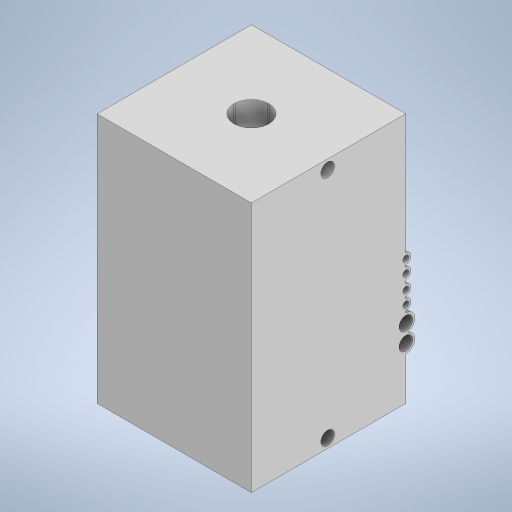
# Autodesk Inventor part: LightSensorHousing
Saved by Autodesk Inventor 2023 (Build 270158000, 158)
## iProperties
Created: 2023-07-05
Part Number: LightSensorHousing
Material: Generic
Document SubType Name: Modeling
Designer: efarq
Density: 1 g/cm^3
Appearance: Default
Author: efarq
Autodesk Inventor part; units mm, degrees
ref_plane "YZ Plane" through (0, 0, 0) normal (1, 0, 0) x (0, 1, 0)
ref_plane "XZ Plane" through (0, 0, 0) normal (0, 1, 0) x (-1, 0, 0)
ref_plane "XY Plane" through (0, 0, 0) normal (0, 0, 1) x (1, 0, 0)
sketch "Sketch1" plane through (0, 0, 0) normal (0, 0, 1) x (1, 0, 0)
  line L0 (-25.4, -41.275) -> (25.4, -41.275)
  line L1 (25.4, -41.275) -> (25.4, 41.275)
  line L2 (25.4, 41.275) -> (-25.4, 41.275)
  line L3 (-25.4, 41.275) -> (-25.4, -41.275)
  line L4 (-25.4, -41.275) -> (25.4, 41.275) construction
  line L5 (25.4, -41.275) -> (-25.4, 41.275) construction
  point P0 (0, 0)
  dimension "d0" = 50.8
  dimension "d1" = 82.55
  constraints: 12 end point, 2 midpoint, 2 parallel, 1 horizontal, 1 perpendicular
  measures "d0" distance of L2.end L1.end
  measures "d1" distance of L0.end L1.end
extrude "Extrusion1" add sketch "Sketch1" along normal blind 50.8
sketch "Sketch2" plane through (-25.4, 41.275, 0) normal (0, 1, 0) x (1, 0, 0)
  circle A0 centre (25.4, -25.4) radius 5.715
  line L0 (50.8, 0) -> (0, 0) projected
  point P0 (25.4, 0)
  dimension "d4" = 11.43
  dimension "d5" = 25.4
  constraints: 1 centre point
  measures "d4" diameter of A0
  measures "d5" distance from line of L0 A0.centre
extrude "Extrusion2" cut sketch "Sketch2" against normal blind 33.02
sketch "Sketch3" plane through (0, 0, 0) normal (0, 0, -1) x (-1, 0, 0)
  line L0 (-13.97, 8.255) -> (13.97, 8.255)
  line L1 (13.97, 8.255) -> (13.97, 28.575)
  line L2 (13.97, 28.575) -> (-13.97, 28.575)
  line L3 (-13.97, 28.575) -> (-13.97, 8.255)
  line L4 (-13.97, 8.255) -> (13.97, 28.575) construction
  line L5 (13.97, 8.255) -> (-13.97, 28.575) construction
  line L6 (-25.4, 41.275) -> (25.4, 41.275) projected
  line L7 (25.4, 41.275) -> (25.4, -41.275) projected
  point P0 (0, 0)
  point P1 (0, 18.415)
  dimension "d9" = 27.94
  dimension "d10" = 20.32
  dimension "d11" = 12.7
  dimension "d14" = 25.4
  constraints: 12 end point, 2 midpoint, 2 parallel, 1 horizontal, 1 perpendicular
  measures "d9" distance of L1.end L2.end
  measures "d10" distance of L0.end L1.end
  measures "d11" distance between parallel lines of L2 L6
  measures "d14" distance from line of L7 point (0, 18.415)
extrude "Extrusion3" cut sketch "Sketch3" against normal blind 19.304
sketch "Sketch6" plane through (0, 0, 19.304) normal (0, 0, -1) x (-1, 0, 0)
  line L0 (-13.97, 15.113) -> (-9.144, 15.113)
  line L1 (-9.144, 15.113) -> (-9.144, 21.717)
  line L2 (-9.144, 21.717) -> (-13.97, 21.717)
  line L3 (-13.97, 21.717) -> (-13.97, 15.113)
  line L4 (-13.97, 15.113) -> (-9.144, 21.717) construction
  line L5 (-9.144, 15.113) -> (-13.97, 21.717) construction
  line L6 (13.97, 28.575) -> (13.97, 8.255) projected
  line L7 (9.144, 15.113) -> (13.97, 15.113)
  line L8 (13.97, 15.113) -> (13.97, 21.717)
  line L9 (13.97, 21.717) -> (9.144, 21.717)
  line L10 (9.144, 21.717) -> (9.144, 15.113)
  line L11 (9.144, 15.113) -> (13.97, 21.717) construction
  line L12 (13.97, 15.113) -> (9.144, 21.717) construction
  line L13 (-13.97, 8.255) -> (-13.97, 28.575) projected
  line L14 (-13.97, 28.575) -> (13.97, 28.575) projected
  point P0 (0, 0)
  point P1 (-11.557, 18.415)
  point P2 (11.557, 18.415)
  point P3 (13.97, 15.113)
  dimension "d15" = 6.604
  dimension "d16" = 4.826
  dimension "d17" = 2.413
  dimension "d18" = 4.826
  dimension "d19" = 6.604
  dimension "d21" = 6.858
  dimension "d22" = 6.858
  constraints: 24 end point, 4 midpoint, 4 parallel, 2 horizontal, 2 perpendicular, 1 point on line
  measures "d15" distance of L0.end L1.end
  measures "d16" distance of L1.end L2.end
  measures "d17" distance from line of L13 point (-11.557, 18.415)
  measures "d18" distance of L8.end L9.end
  measures "d19" distance of L9.end L7.start
  measures "d21" distance between parallel lines of L9 L14
  measures "d22" distance between parallel lines of L14 L2
extrude "Extrusion4" cut sketch "Sketch6" against normal blind 4.826
sketch "Sketch7" plane through (0, 0, 19.304) normal (0, 0, -1) x (-1, 0, 0)
  line L0 (-2.3813, 16.0401) -> (2.3813, 16.0401)
  line L1 (2.3813, 16.0401) -> (2.3812, 20.8026)
  line L2 (2.3812, 20.8026) -> (-2.3813, 20.8026)
  line L3 (-2.3813, 20.8026) -> (-2.3813, 16.0401)
  line L4 (-2.3813, 16.0401) -> (2.3812, 20.8026) construction
  line L5 (2.3813, 16.0401) -> (-2.3813, 20.8026) construction
  line L6 (9.144, 15.113) -> (9.144, 21.717) projected
  line L7 (-13.97, 28.575) -> (13.97, 28.575) projected
  point P0 (0, 0)
  point P1 (0, 18.4213)
  point P2 (0, 20.8026)
  dimension "d25" = 4.7625
  dimension "d26" = 9.144
  dimension "d27" = 4.7625
  dimension "d29" = 7.7724
  constraints: 12 end point, 3 midpoint, 2 parallel, 1 horizontal, 1 perpendicular
  measures "d25" distance of L1.end L2.end
  measures "d26" distance from line of L6 point (0, 18.421)
  measures "d27" distance of L2.end L0.start
  measures "d29" distance from line of point (0, 20.803) L7
extrude "Extrusion5" cut sketch "Sketch7" against normal blind 4.826
sketch "Sketch8" plane through (-25.4, -41.275, 0) normal (-1, 0, 0) x (0, 0, 1)
  line L0 (15.24, 11.43) -> (35.56, 11.43)
  line L1 (35.56, 11.43) -> (35.56, 57.15)
  line L2 (35.56, 57.15) -> (15.24, 57.15)
  line L3 (15.24, 57.15) -> (15.24, 11.43)
  line L4 (15.24, 11.43) -> (35.56, 57.15) construction
  line L5 (35.56, 11.43) -> (15.24, 57.15) construction
  line L6 (50.8, 82.55) -> (50.8, 0) projected
  line L7 (0, 82.55) -> (50.8, 82.55) projected
  point P0 (0, 41.275)
  point P1 (25.4, 34.29)
  dimension "d32" = 45.72
  dimension "d33" = 20.32
  dimension "d34" = 25.4
  dimension "d35" = 25.4
  constraints: 12 end point, 2 midpoint, 2 parallel, 1 horizontal, 1 perpendicular
  measures "d32" distance of L0.end L1.end
  measures "d33" distance of L0.start L0.end
  measures "d34" distance from line of L6 point (25.4, 34.29)
  measures "d35" distance between parallel lines of L7 L2
extrude "Extrusion6" cut sketch "Sketch8" against normal blind 10.16
sketch "Sketch11" plane through (-25.4, -41.275, 0) normal (-1, 0, 0) x (0, 0, 1)
  circle A0 centre (27.4828, 60.96) radius 3.302
  line L0 (0, 82.55) -> (50.8, 82.55) projected
  line L1 (50.8, 82.55) -> (50.8, 0) projected
  point P0 (0, 41.275)
  dimension "d43" = 6.604
  dimension "d44" = 21.59
  dimension "d45" = 23.3172
  constraints: 1 centre point
  measures "d43" diameter of A0
  measures "d44" distance from line of A0.centre L0
  measures "d45" distance from line of L1 A0.centre
extrude "Extrusion7" cut sketch "Sketch11" against normal blind 25.4
sketch "Sketch14" plane through (-25.4, 41.275, 0) normal (0, 1, 0) x (1, 0, 0)
  line L0 (19.685, -31.115) -> (31.115, -31.115)
  line L1 (31.115, -31.115) -> (31.115, -19.685)
  line L2 (31.115, -19.685) -> (19.685, -19.685)
  line L3 (19.685, -19.685) -> (19.685, -31.115)
  circle A0 centre (25.4, -25.4) radius 5.715 projected
  line L4 (19.685, -31.115) -> (31.115, -19.685) construction
  line L5 (31.115, -31.115) -> (19.685, -19.685) construction
  point P0 (25.4, 0)
  constraints: 12 end point, 2 midpoint, 2 parallel, 1 horizontal, 1 perpendicular
extrude "Extrusion8" cut sketch "Sketch14" against normal blind 33.02
sketch "Sketch15" plane through (-25.4, 41.275, 0) normal (0, 1, 0) x (1, 0, 0)
  circle A0 centre (25.4, -25.4) radius 5.725
  line L0 (31.115, -19.685) -> (31.115, -31.115) projected
  line L1 (19.685, -19.685) -> (31.115, -19.685)
  line L2 (31.115, -19.685) -> (31.115, -31.115)
  line L3 (31.115, -31.115) -> (19.685, -31.115)
  line L4 (19.685, -31.115) -> (19.685, -19.685)
  line L5 (19.685, -19.685) -> (31.115, -31.115) construction
  line L6 (31.115, -19.685) -> (19.685, -31.115) construction
  point P0 (25.4, 0)
  point P1 (19.685, -25.0617)
  point P2 (25.0617, -19.685)
  point P3 (25.7383, -19.685)
  point P4 (31.115, -25.0617)
  point P5 (19.685, -25.7383)
  point P6 (25.0617, -31.115)
  point P7 (25.7383, -31.115)
  point P8 (31.115, -25.7383)
  constraints: 12 end point, 2 midpoint, 2 parallel, 1 centre point, 1 horizontal, 1 perpendicular
extrude "Extrusion9" add sketch "Sketch15" against normal blind 10.16 contours A0 L1 L0 | L0 L3 A0 | A0 L4 L1 | L3 L4 A0
sketch "Sketch16" plane through (-25.4, 15.875, 15.24) normal (0, -1, 0) x (1, 0, 0)
  circle A0 centre (2.2186, 12.8252) radius 0.4886
  circle A1 centre (2.2186, 11.3059) radius 0.4826
  line L0 (11.43, 4.064) -> (11.43, 8.89) projected
  point P0 (25.4, -15.24)
  dimension "d57" = 0.9772
  dimension "d59" = 0.9652
  constraints: 2 centre point
  measures "d57" diameter of A0
  measures "d59" diameter of A1
extrude "Extrusion10" cut sketch "Sketch16" against normal blind 2.54
sketch "Sketch17" plane through (25.4, -41.275, 0) normal (1, 0, 0) x (0, 0, -1)
  line L0 (-25.7383, 82.55) -> (-25.7383, 72.39) projected
  circle A0 centre (-25.7383, 79.502) radius 2.2209
  circle A1 centre (-25.7383, 3.048) radius 2.2225
  line L1 (0, 82.55) -> (-50.8, 82.55) projected
  line L2 (0, 0) -> (-50.8, 0) projected
  point P0 (0, 41.275)
  dimension "d62" = 4.4418
  dimension "d63" = 4.445
  dimension "d64" = 3.048
  dimension "d65" = 3.048
  constraints: 2 centre point, 1 point on line
  measures "d62" diameter of A0
  measures "d63" diameter of A1
  measures "d64" distance from line of L1 A0.centre
  measures "d65" distance from line of L2 A1.centre
extrude "Extrusion11" cut sketch "Sketch17" against normal blind 7
sketch "Sketch18" plane through (25.4, -41.275, 0) normal (1, 0, 0) x (0, 0, -1)
  line L0 (0, 0) -> (0, 82.55) projected
  circle A0 centre (0, 41.275) radius 1.75
  point P0 (0, 41.275)
  dimension "d71" = 3.5
  constraints: 1 centre point, 1 coincident, 1 midpoint
  measures "d71" diameter of A0
extrude "Extrusion12" add sketch "Sketch18" against normal blind 16.5
sketch "Sketch19" plane through (-13.97, 8.255, 0) normal (0, 1, 0) x (1, 0, 0)
  line L0 (0, 0) -> (27.94, 0) projected
  circle A0 centre (24.62, 0) radius 1.75
  line L1 (22.87, 1.75) -> (22.87, 0) projected
  point P0 (13.97, 0)
  dimension "d77" = 3.5
  dimension "d78" = 1.75
  constraints: 1 centre point, 1 point on line
  measures "d77" diameter of A0
  measures "d78" distance from line of L1 A0.centre
extrude "Extrusion13" add sketch "Sketch19" against normal blind 8
sketch "Sketch20" plane through (25.4, -41.275, 50.8) normal (1, 0, 0) x (0, 0, -1)
  circle A0 centre (50.8, 41.275) radius 1
  dimension "d81" = 2
  constraints: 1 centre point, 1 coincident
  measures "d81" diameter of A0
extrude "Extrusion14" cut sketch "Sketch20" against normal blind 16
sketch "Sketch21" plane through (-13.97, 8.255, 19.304) normal (0, 1, 0) x (1, 0, 0)
  circle A0 centre (24.6331, 19.304) radius 1
  arc A1 (26.37, 19.304) -> (22.87, 19.304) centre (24.62, 19.304) ccw projected
  point P0 (13.97, 19.304)
  dimension "d84" = 2
  constraints: 1 centre point
  measures "d84" diameter of A0
extrude "Extrusion15" cut sketch "Sketch21" against normal blind 8.5
sketch "Sketch22" plane through (25.4, -41.275, 50.8) normal (1, 0, 0) x (0, 0, -1)
  line L0 (50.8, 82.55) -> (50.8, 0) projected
  circle A0 centre (50.8, 37.084) radius 1.75
  point P0 (50.8, 41.275)
  point P1 (50.8, 41.275)
  dimension "d88" = 3.5
  dimension "d89" = 4.191
  constraints: 1 centre point, 1 midpoint, 1 point on line
  measures "d88" diameter of A0
  measures "d89" distance of A0.centre point (50.8, 41.275)
extrude "Extrusion16" add sketch "Sketch22" against normal blind 20.75
sketch "Sketch23" plane through (-13.97, 8.255, 19.304) normal (0, 1, 0) x (1, 0, 0)
  line L0 (0, 19.304) -> (22.87, 19.304) projected
  circle A0 centre (20.429, 19.304) radius 1.75
  arc A1 (26.37, 19.304) -> (22.87, 19.304) centre (24.62, 19.304) ccw projected
  point P0 (13.97, 19.304)
  dimension "d92" = 3.5
  dimension "d93" = 4.191
  constraints: 1 centre point, 1 point on line
  measures "d92" diameter of A0
  measures "d93" distance of A1.centre A0.centre
extrude "Extrusion17" add sketch "Sketch23" against normal blind 12
sketch "Sketch24" plane through (-13.97, 8.255, 19.304) normal (0, 1, 0) x (1, 0, 0)
  circle A0 centre (20.4444, 19.304) radius 1
  arc A1 (22.179, 19.304) -> (18.679, 19.304) centre (20.429, 19.304) ccw projected
  point P0 (13.97, 19.304)
  dimension "d96" = 2
  dimension "d97" = 0.0154
  constraints: 1 centre point
  measures "d96" diameter of A0
  measures "d97" distance of A0.centre A1.centre
extrude "Extrusion18" cut sketch "Sketch24" against normal blind 13
sketch "Sketch25" plane through (25.4, -41.275, 50.8) normal (1, 0, 0) x (0, 0, -1)
  line L0 (50.8, 38.834) -> (50.8, 35.334) projected
  circle A0 centre (50.8, 37.084) radius 1
  point P0 (50.8, 41.275)
  dimension "d100" = 2
  constraints: 1 centre point, 1 midpoint
  measures "d100" diameter of A0
extrude "Extrusion19" cut sketch "Sketch25" against normal blind 20
sketch "Sketch26" plane through (25.4, -41.275, 50.8) normal (1, 0, 0) x (0, 0, -1)
  line L0 (50.8, 82.55) -> (50.8, 0) projected
  circle A0 centre (50.8, 32.3936) radius 1.75
  point P0 (50.8, 41.275)
  dimension "d103" = 3.5
  constraints: 1 centre point, 1 point on line
  measures "d103" diameter of A0
extrude "Extrusion20" add sketch "Sketch26" against normal blind 30
sketch "Sketch27" plane through (-13.97, 8.255, 19.304) normal (0, 1, 0) x (1, 0, 0)
  line L0 (0, 19.304) -> (18.679, 19.304) projected
  circle A0 centre (11.12, 19.304) radius 1.75
  line L1 (9.37, 21.054) -> (9.37, 19.304) projected
  point P0 (13.97, 19.304)
  dimension "d106" = 3.5
  dimension "d107" = 1.75
  constraints: 1 centre point, 1 point on line
  measures "d106" diameter of A0
  measures "d107" distance from line of L1 A0.centre
extrude "Extrusion21" add sketch "Sketch27" against normal blind 17
sketch "Sketch28" plane through (-13.97, 8.255, 19.304) normal (0, 1, 0) x (1, 0, 0)
  circle A0 centre (11.1074, 19.304) radius 1
  point P0 (13.97, 19.304)
  dimension "d110" = 2
  constraints: 1 centre point
  measures "d110" diameter of A0
extrude "Extrusion22" cut sketch "Sketch28" against normal blind 17
sketch "Sketch30" plane through (25.4, -41.275, 50.8) normal (1, 0, 0) x (0, 0, -1)
  line L0 (50.8, 82.55) -> (50.8, 0) projected
  circle A0 centre (50.8, 32.3913) radius 1
  point P0 (50.8, 41.275)
  dimension "d113" = 2
  constraints: 1 centre point, 1 point on line
  measures "d113" diameter of A0
extrude "Extrusion23" cut sketch "Sketch30" against normal blind 29.5
sketch "Sketch31" plane through (25.4, -41.275, 50.8) normal (1, 0, 0) x (0, 0, -1)
  line L0 (50.8, 0) -> (50.8, 30.6436) projected
  circle A0 centre (50.8, 28.2026) radius 1.75
  line L1 (50.8, 34.1436) -> (50.8, 30.6436) projected
  point P0 (50.8, 41.275)
  point P1 (50.8, 32.3936)
  dimension "d116" = 3.5
  dimension "d117" = 4.191
  constraints: 1 centre point, 1 midpoint, 1 point on line
  measures "d116" diameter of A0
  measures "d117" distance of point (50.8, 32.394) A0.centre
extrude "Extrusion24" add sketch "Sketch31" against normal blind 34.25
sketch "Sketch32" plane through (-13.97, 8.255, 19.304) normal (0, 1, 0) x (1, 0, 0)
  line L0 (0, 19.304) -> (9.37, 19.304) projected
  circle A0 centre (6.9164, 19.304) radius 1.75
  circle A1 centre (11.1074, 19.304) radius 1 projected
  point P0 (13.97, 19.304)
  dimension "d120" = 3.5
  dimension "d121" = 4.191
  constraints: 1 centre point, 1 point on line
  measures "d120" diameter of A0
  measures "d121" distance of A0.centre A1.centre
extrude "Extrusion25" add sketch "Sketch32" against normal blind 21 contours A0 L0 | L0 A0
sketch "Sketch33" plane through (25.4, -41.275, 50.8) normal (1, 0, 0) x (0, 0, -1)
  line L0 (50.8, 29.9526) -> (50.8, 26.4526) projected
  circle A0 centre (50.8, 28.2026) radius 1
  point P0 (50.8, 41.275)
  dimension "d124" = 2
  constraints: 1 centre point, 1 midpoint
  measures "d124" diameter of A0
extrude "Extrusion26" cut sketch "Sketch33" against normal blind 33
sketch "Sketch34" plane through (-13.97, 8.255, 19.304) normal (0, 1, 0) x (1, 0, 0)
  arc A0 (8.6664, 19.304) -> (5.1664, 19.304) centre (6.9164, 19.304) ccw projected
  circle A1 centre (6.9164, 19.304) radius 1
  point P0 (13.97, 19.304)
  dimension "d127" = 2
  constraints: 1 centre point, 1 coincident
  measures "d127" diameter of A1
extrude "Extrusion27" cut sketch "Sketch34" against normal blind 22.5
sketch "Sketch35" plane through (25.4, -41.275, 50.8) normal (1, 0, 0) x (0, 0, -1)
  line L0 (50.8, 0) -> (50.8, 26.4526) projected
  circle A0 centre (50.8, 22.8686) radius 3
  circle A1 centre (50.8, 28.2026) radius 1 projected
  point P0 (50.8, 41.275)
  dimension "d130" = 6
  dimension "d131" = 5.334
  constraints: 1 centre point, 1 point on line
  measures "d130" diameter of A0
  measures "d131" distance of A0.centre A1.centre
extrude "Extrusion28" add sketch "Sketch35" against normal blind 45 contours A0 L0 | L0 A0
sketch "Sketch36" plane through (25.4, -41.275, 50.8) normal (1, 0, 0) x (0, 0, -1)
  line L0 (50.8, 82.55) -> (50.8, 0) projected
  circle A0 centre (50.8, 17.0266) radius 3
  arc A1 (50.8, 19.8686) -> (50.8, 25.8686) centre (50.8, 22.8686) ccw projected
  point P0 (50.8, 41.275)
  dimension "d134" = 6
  dimension "d135" = 5.842
  constraints: 1 centre point, 1 point on line
  measures "d134" diameter of A0
  measures "d135" distance of A0.centre A1.centre
extrude "Extrusion29" add sketch "Sketch36" against normal blind 45 contours A0 A1 L0 | L0 A0 | A0 L0 A1 picked at (50.8766, 19.971) picked at (51.0225, 15.999)
sketch "Sketch38" plane through (25.4, -41.275, 50.8) normal (1, 0, 0) x (0, 0, -1)
  line L0 (50.8, 82.55) -> (50.8, 0) projected
  circle A0 centre (50.8, 22.882) radius 2.25
  circle A1 centre (50.8, 17.1667) radius 2.25
  point P0 (50.8, 41.275)
  dimension "d139" = 4.5
  dimension "d140" = 4.5
  constraints: 2 centre point
  measures "d139" diameter of A0
  measures "d140" diameter of A1
extrude "Extrusion30" cut sketch "Sketch38" against normal blind 44
sketch "Sketch39" plane through (-25.4, -29.845, 15.24) normal (0, 0, 1) x (1, 0, 0)
  line L0 (8.5111, 2.5959) -> (4.7011, 2.5959)
  line L1 (4.7011, 2.5959) -> (4.7011, 13.9243)
  line L2 (4.7011, 13.9243) -> (8.5111, 13.9243)
  line L3 (8.5111, 13.9243) -> (8.5111, 2.5959)
  line L4 (8.5111, -0.4043) -> (7.0851, 7.4931) construction
  line L5 (-0.3554, -0.4043) -> (5.3241, 7.2919) construction
  point P0 (25.4, 29.845)
  point P1 (7.7981, 3.5444)
  point P2 (0, -11.43)
  dimension "d145" = 11.3284
  dimension "d146" = 3.81
  dimension "d147" = 14.0259
  constraints: 12 end point, 2 parallel, 1 horizontal, 1 midpoint, 1 perpendicular
  measures "d145" distance of L2.end L0.start
  measures "d146" distance of L1.end L2.end
  measures "d147" distance from line of point (0, -11.43) L0
extrude "Extrusion31" cut sketch "Sketch39" against normal blind 16
body "Solid1"
